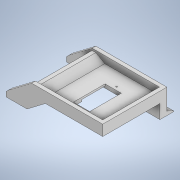
# Autodesk Inventor part: mount_for_plugs
Saved by Autodesk Inventor 2022 (Build 260153000, 153)
## iProperties
Created: 2022-01-23
Part Number: mount_for_plugs
Material: Generic
Document SubType Name: Modeling
Designer: kylem
Density: 1 g/cm^3
Appearance: Default
Author: kylem
Autodesk Inventor part; units mm, degrees
ref_plane "YZ Plane" through (0, 0, 0) normal (1, 0, 0) x (0, 1, 0)
ref_plane "XZ Plane" through (0, 0, 0) normal (0, 1, 0) x (-1, 0, 0)
sketch "Sketch1" plane through (0, 0, 0) normal (0, 1, 0) x (-1, 0, 0)
  line L0 (0, 0) -> (159.6, 0)
  line L1 (159.6, 46) -> (159.6, 118)
  line L2 (159.6, 118) -> (0, 118)
  line L3 (0, 118) -> (0, 0)
  line L4 (159.6, 118) -> (159.6, 46)
  line L5 (0, 0) -> (113, 0)
  line L6 (113, 0) -> (159.6, 46)
  line L7 (159.6, 118) -> (167.6, 118)
  line L8 (167.6, 118) -> (167.6, 46)
  line L9 (167.6, 46) -> (159.6, 46)
  line L10 (159.6, 46) -> (159.6, 118)
  line L11 (113, 0) -> (0, 0)
  line L12 (0, 0) -> (0, -8)
  line L13 (0, -8) -> (113, -8)
  line L14 (113, -8) -> (113, 0)
  line L15 (0, 0) -> (0, 10)
  line L16 (0, 10) -> (9, 10)
  circle A0 centre (9, 10) radius 2.25
  line L17 (159.6, 118) -> (159.6, 89)
  line L18 (159.6, 89) -> (149.6, 89)
  circle A1 centre (149.6, 89) radius 2.25
  line L19 (159.6, 118) -> (159.6, 0)
  dimension "d0" = 159.6
  dimension "d2" = 72
  dimension "d3" = 113
  dimension "d4" = 8
  dimension "d5" = 8
  dimension "d6" = 10
  dimension "d7" = 9
  dimension "d8" = 4.5
  dimension "d9" = 29
  dimension "d10" = 10
  dimension "d11" = 4.5
  dimension "d14" = 118
  constraints: 40 end point, 6 parallel, 5 perpendicular, 3 horizontal, 3 point on line, 2 centre point, 2 coincident, 1 collinear
  measures "d0" distance of L2.end L1.end
  measures "d2" distance of L1.start L1.end
  measures "d3" distance of L0.start L5.end
  measures "d4" distance of L1.start L8.end
  measures "d5" distance of L12.end L11.end
  measures "d6" distance of L11.end L15.end
  measures "d7" distance of L15.end L16.end
  measures "d8" diameter of A0
  measures "d9" distance of L1.end L17.end
  measures "d10" distance of L17.end L18.end
  measures "d11" diameter of A1
  measures "d14" distance of L1.end L0.end
extrude "Extrusion2" add sketch "Sketch1" along normal blind 8 contours L3 L2 L1 L6 L0 | L0 L14 L13 L12 | L1 L7 L8 L9
sketch "Sketch2" plane through (0, 8, 0) normal (0, 1, 0) x (1, 0, 0)
  line L0 (-113, 8) -> (-113, 0) projected
  line L1 (-159.6, -46) -> (-113, 0)
  line L2 (-113, 0) -> (-94.4074, 18.3532)
  line L3 (-113, 0) -> (-159.6, -46) projected
  line L4 (-113, 0) -> (-159.6, -46)
  line L5 (-159.6, -46) -> (-175.759, -61.951)
  line L6 (-175.759, -61.951) -> (-174.3006, -39.4963)
  line L7 (-174.3006, -39.4963) -> (-106.8014, 20.2158)
  line L8 (-106.8014, 20.2158) -> (-94.4074, 18.3532)
  point P0 (0, 0)
  constraints: 14 end point, 2 point on line, 1 collinear
extrude "Extrusion3" cut sketch "Sketch2" against normal blind 10
sketch "Sketch3" plane through (0, 0, 0) normal (0, -1, 0) x (1, 0, 0)
  line L0 (-167.6, 118) -> (0, 118) projected
  line L1 (-167.6, 118) -> (-167.6, 92.4)
  line L2 (-167.6, 53.897) -> (-167.6, 118) projected
  line L3 (-167.6, 92.4) -> (-128, 92.4)
  line L4 (-128, 92.4) -> (-120.5, 92.4)
  line L5 (-120.5, 92.4) -> (-120.5, 88.9)
  line L6 (-120.5, 88.9) -> (-128, 88.9)
  line L7 (-128, 88.9) -> (-128, 92.4)
  line L8 (-120.5, 88.9) -> (-120.5, 56.15)
  line L9 (-120.5, 88.9) -> (-87.75, 88.9) construction
  circle A0 centre (-120.5, 88.9) radius 1.15
  circle A1 centre (-120.5, 56.15) radius 1.15
  line L10 (-120.5, 88.9) -> (-120.5, 90.9)
  line L11 (-120.5, 88.9) -> (-120.5, 85.9)
  line L12 (-120.5, 56.15) -> (-120.5, 59.15)
  line L13 (-120.5, 59.15) -> (-115, 59.15)
  line L14 (-120.5, 85.9) -> (-126, 85.9)
  line L15 (-126, 85.9) -> (-115, 85.9)
  line L16 (-115, 85.9) -> (-115, 59.15)
  line L17 (-115, 59.15) -> (-126, 59.15)
  line L18 (-126, 59.15) -> (-126, 85.9)
  point P0 (0, 0)
  dimension "d19" = 25.6
  dimension "d20" = 39.6
  dimension "d21" = 7.5
  dimension "d22" = 3.5
  dimension "d23" = 32.75
  dimension "d24" = 90
  dimension "d25" = 2.3
  dimension "d26" = 2.3
  dimension "d29" = 2
  dimension "d30" = 3
  dimension "d31" = 3
  dimension "d32" = 5.5
  dimension "d33" = 5.5
  constraints: 34 end point, 5 horizontal, 4 parallel, 4 perpendicular, 4 point on line, 2 centre point, 2 coincident, 1 vertical
  measures "d19" distance of L0.start L1.end
  measures "d20" distance of L1.end L3.end
  measures "d21" distance of L5.end L6.end
  measures "d22" distance of L4.end L5.end
  measures "d23" distance of L5.end L8.end
  measures "d24" angle of L8 L9
  measures "d25" diameter of A0
  measures "d26" diameter of A1
  measures "d29" distance of L10.start L10.end
  measures "d30" distance of L10.start L11.end
  measures "d31" distance of L12.start L12.end
  measures "d32" distance of L12.end L13.end
  measures "d33" distance of L11.end L14.end
extrude "Extrusion4" cut sketch "Sketch3" against normal blind 5 contours A0 L5 L6 | L6 L8 A0 | A0 L8 L5 | A1
sketch "Sketch5" plane through (0, 8, 0) normal (0, 1, 0) x (1, 0, 0)
  circle A0 centre (-9, -10) radius 2.25 projected
  circle A1 centre (-149.6, -89) radius 2.25 projected
  line L0 (-9, -10) -> (-149.6, -89)
  line L1 (-149.6, -89) -> (-116.8523, -147.2827)
  line L2 (-116.8523, -147.2827) -> (-175.4275, -43.0335)
  line L3 (-149.6, -89) -> (-9, -10)
  line L4 (-79.3, -49.5) -> (-9, -10)
  line L5 (-149.6, -89) -> (-144.7015, -97.7181)
  line L6 (-116.8523, -147.2827) -> (-175.4275, -43.0335)
  line L7 (-175.4275, -43.0335) -> (-34.8275, 35.9665)
  line L8 (-34.8275, 35.9665) -> (23.7477, -68.2827)
  line L9 (23.7477, -68.2827) -> (-116.8523, -147.2827)
  circle A2 centre (-9, -10) radius 4.5 projected
  line L10 (-9, -10) -> (-4.1015, -18.7181)
  line L11 (-4.1015, -18.7181) -> (-1.6523, -23.0771)
  line L12 (-1.6523, -23.0771) -> (8.1447, -40.5133)
  line L13 (8.1447, -40.5133) -> (10.594, -44.8723)
  line L14 (-144.7015, -97.7181) -> (-142.2523, -102.0771)
  line L15 (-142.2523, -102.0771) -> (-132.4553, -119.5133)
  line L16 (-132.4553, -119.5133) -> (-130.006, -123.8723)
  line L17 (-149.6, -89) -> (-154.4985, -80.2819)
  line L18 (-154.4985, -80.2819) -> (-156.9477, -75.9229)
  line L19 (-9, -10) -> (-13.8985, -1.2819)
  line L20 (-13.8985, -1.2819) -> (-16.3477, 3.0771)
  line L21 (-167.6, -53.897) -> (-167.6, -118) projected
  line L22 (-167.6, -118) -> (0, -118)
  line L23 (0, -118) -> (0, 8)
  line L24 (0, 8) -> (-167.6, 8)
  line L25 (-167.6, 8) -> (-167.6, -118)
  line L26 (-16.3477, 3.0771) -> (-156.9477, -75.9229)
  line L27 (-154.4985, -80.2819) -> (-13.8985, -1.2819)
  line L28 (-4.1015, -18.7181) -> (-144.7015, -97.7181)
  line L29 (-142.2523, -102.0771) -> (-1.6523, -23.0771)
  line L30 (8.1447, -40.5133) -> (-132.4553, -119.5133)
  line L31 (-130.006, -123.8723) -> (10.594, -44.8723)
  line L32 (-4.1015, -18.7181) -> (7.818, -12.0208)
  line L33 (-1.6523, -23.0771) -> (4.3075, -19.7285)
  line L34 (-13.8985, -1.2819) -> (7.818, 10.9201)
  line L35 (-16.3477, 3.0771) -> (3.62, 14.2965)
  line L36 (-144.7015, -97.7181) -> (-142.2523, -102.0771)
  line L37 (-142.2523, -102.0771) -> (-178.8351, -122.6322)
  line L38 (-178.8351, -122.6322) -> (-181.2843, -118.2731)
  line L39 (-181.2843, -118.2731) -> (-144.7015, -97.7181)
  line L40 (-154.4985, -80.2819) -> (-156.9477, -75.9229)
  line L41 (-156.9477, -75.9229) -> (-183.573, -90.883)
  line L42 (-183.573, -90.883) -> (-181.1237, -95.242)
  line L43 (-181.1237, -95.242) -> (-154.4985, -80.2819)
  line L44 (0, 8) -> (-104.8957, 8) projected
  line L45 (0, 8) -> (-5, 8)
  line L46 (-5, 8) -> (-5, 3)
  line L47 (-5, 3) -> (0, 3)
  line L48 (0, 3) -> (0, 8)
  line L49 (-104.8957, 8) -> (-167.6, -53.897) projected
  line L50 (-104.8957, 8) -> (-167.6, -53.897)
  line L51 (-167.6, -53.897) -> (-164.0874, -57.4554)
  line L52 (-164.0874, -57.4554) -> (-101.3831, 4.4416)
  line L53 (-101.3831, 4.4416) -> (-104.8957, 8)
  line L54 (0, -118) -> (0, 8) projected
  line L55 (0, 3) -> (0, 8)
  line L56 (0, 8) -> (-113.2487, 8)
  line L57 (-113.2487, 8) -> (-113.2487, 3)
  line L58 (-113.2487, 3) -> (0, 3)
  line L59 (-5, 8) -> (0, 8)
  line L60 (0, 8) -> (0, -118)
  line L61 (0, -118) -> (-5, -118)
  line L62 (-5, -118) -> (-5, 8)
  line L63 (-167.6, -118) -> (0, -118) projected
  line L64 (-167.6, -118) -> (-162.6, -118)
  line L65 (-162.6, -118) -> (-162.6, -39.4397)
  line L66 (-162.6, -39.4397) -> (-167.6, -39.4397)
  line L67 (-167.6, -39.4397) -> (-167.6, -118)
  line L68 (-167.6, -118) -> (0, -118) projected
  line L69 (0, -118) -> (-186.0038, -118)
  line L70 (-186.0038, -118) -> (-186.0038, -113)
  line L71 (-186.0038, -113) -> (0, -113)
  line L72 (0, -113) -> (0, -118)
  point P0 (0, 0)
  point P1 (-162.6, -107.7748)
  point P2 (-162.6, -84.834)
  point P3 (-6.2777, 3)
  point P4 (-5, -7.9384)
  point P5 (-5, -12.0616)
  point P6 (-5, -19.2229)
  point P7 (-5, -24.9581)
  point P8 (-5, -47.899)
  point P9 (-120.8633, -113)
  point P10 (-161.6922, -113)
  point P11 (-162.6, -113.51)
  point P12 (-162.6, -113)
  point P13 (-5, -113)
  point P14 (-110.6561, -113)
  point P15 (-5, -53.6342)
  point P16 (-162.6, -79.0988)
  point P17 (-162.6, -55.9871)
  point P18 (-102.8435, 3)
  point P19 (-16.485, 3)
  point P20 (-16.3044, 3)
  dimension "d45" = 10
  dimension "d46" = 10
  dimension "d47" = 5
  dimension "d48" = 20
  dimension "d49" = 5
  dimension "d50" = 5
  dimension "d51" = 20
  dimension "d52" = 5
  dimension "d53" = 10
  dimension "d54" = 5
  dimension "d55" = 10
  dimension "d56" = 5
  dimension "d57" = 5
  dimension "d58" = 5
  dimension "d59" = 5
  dimension "d60" = 5
  dimension "d61" = 5
  constraints: 134 end point, 20 parallel, 14 point on line, 13 perpendicular, 7 collinear, 3 horizontal, 1 midpoint
  measures "d45" distance of L0.end L5.end
  measures "d46" distance of L10.start L10.end
  measures "d47" distance of L10.end L11.end
  measures "d48" distance of L11.end L12.end
  measures "d49" distance of L12.end L13.end
  measures "d50" distance of L5.end L14.end
  measures "d51" distance of L14.end L15.end
  measures "d52" distance of L15.end L16.end
  measures "d53" distance of L0.end L17.end
  measures "d54" distance of L17.end L18.end
  measures "d55" distance of L10.start L19.end
  measures "d56" distance of L19.end L20.end
  measures "d57" distance of L47.end L46.end
  measures "d58" distance of L46.end L45.end
  measures "d59" distance of L51.end L21.start
  measures "d60" distance of L66.end L65.end
  measures "d61" distance of L69.end L70.end
extrude "Extrusion7" cut sketch "Sketch3" against normal blind 7 contours L15 L16 L13 L8 | L8 L17 L18 L14
sketch "Sketch7" plane through (0, 0, 0) normal (0, -1, 0) x (1, 0, 0)
  line L0 (-167.6, 118) -> (0, 118) projected
  line L1 (0, 118) -> (-70, 118)
  line L2 (-70, 118) -> (-70, 100.4)
  line L3 (-70, 100.4) -> (-70, 18)
  circle A0 centre (-70, 100.4) radius 1.5
  circle A1 centre (-70, 18) radius 1.5
  point P0 (0, 0)
  dimension "d66" = 70
  dimension "d67" = 17.6
  dimension "d68" = 82.4
  dimension "d69" = 3
  dimension "d70" = 3
  constraints: 6 end point, 2 centre point, 2 coincident, 1 perpendicular, 1 point on line, 1 vertical
  measures "d66" distance of L0.end L1.end
  measures "d67" distance of L1.end L2.end
  measures "d68" distance of L2.end L3.end
  measures "d69" diameter of A0
  measures "d70" diameter of A1
extrude "Extrusion8" cut sketch "Sketch7" against normal blind 30
sketch "Sketch8" plane through (0, 0, 0) normal (0, -1, 0) x (1, 0, 0)
  circle A0 centre (-70, 100.4) radius 1.5 projected
  line L0 (-70, 100.4) -> (-70, 93.4)
  line L1 (-70, 93.4) -> (-52.5, 93.4)
  line L2 (-52.5, 93.4) -> (-87.5, 93.4)
  line L3 (-87.5, 93.4) -> (-87.5, 25.4)
  line L4 (-87.5, 25.4) -> (-52.5, 25.4)
  line L5 (-52.5, 25.4) -> (-52.5, 93.4)
  point P0 (0, 0)
  dimension "d73" = 7
  dimension "d74" = 17.5
  dimension "d75" = 35
  dimension "d76" = 68
  constraints: 12 end point, 2 horizontal, 2 parallel, 1 perpendicular, 1 vertical
  measures "d73" distance of L0.start L0.end
  measures "d74" distance of L0.end L1.end
  measures "d75" distance of L4.end L3.end
  measures "d76" distance of L3.end L2.end
extrude "Extrusion9" cut sketch "Sketch8" against normal blind 23 contours L1 L5 L4 L3 L2
extrude "Extrusion10" add sketch "Sketch5" along normal blind 15 contours L62 L47 L23 L32 L8 A2 | L8 L28 L62 | L8 L35 L24 L46 L34 L58 | L34 L46 L58 | L46 L34 L23 L47 | L32 L23 L33 L8 | L8 L29 L62 L28 | L26 L58 L7 L24 L8 | L8 L24 L35 | L65 L39 L21 L43 | L43 L21 L41 L65 | L46 L24 L23 L34 | L33 L23 L8 | L8 L23 L30 L62 L29 | L58 L52 L53 L24 L7 | L65 L41 L21 L2 | L2 L21 L51 L52 L65 | L65 L71 L21 L39 | L30 L23 L31 L62 | L52 L65 L49 L7 | L7 L49 L58 L52 | L58 L49 L53 L52 | L52 L51 L49 L65 | L71 L37 L65 | L65 L37 L21 L71 | L71 L30 L22 L1 | L1 L22 L65 L37 L71 | L71 L31 L22 L30 | L31 L23 L9 L62 | L65 L22 L21 L37 | L71 L9 L22 L31 | L9 L23 L71 L62 | L71 L62 L22 L9 | L71 L23 L22 L62
sketch "Sketch10" plane through (0, 0, 0) normal (0, -1, 0) x (1, 0, 0)
  line L0 (-52.5, 93.4) -> (-87.5, 93.4) projected
  line L1 (-70, 93.4) -> (-42.5, 93.4)
  line L2 (-42.5, 93.4) -> (-42.5, 75.4)
  line L3 (-42.5, 75.4) -> (-42.5, 25.4)
  line L4 (-42.5, 75.4) -> (-97.5, 75.4)
  line L5 (-97.5, 75.4) -> (-97.5, 25.4)
  line L6 (-97.5, 25.4) -> (-42.5, 25.4)
  line L7 (-42.5, 25.4) -> (-42.5, 75.4)
  point P0 (0, 0)
  point P1 (-42.5, 25.4)
  dimension "d81" = 27.5
  dimension "d82" = 18
  dimension "d83" = 50
  dimension "d84" = 55
  dimension "d87" = 50
  constraints: 14 end point, 2 parallel, 2 perpendicular, 1 collinear, 1 horizontal, 1 midpoint, 1 point on line
  measures "d81" distance of L1.start L1.end
  measures "d82" distance of L1.end L2.end
  measures "d83" distance of L2.end L3.end
  measures "d84" distance of L6.end L5.end
  measures "d87" distance of L4.end L5.end
extrude "Extrusion11" cut sketch "Sketch10" against normal blind 4
sketch "Sketch11" plane through (0, 8, 0) normal (0, 1, 0) x (1, 0, 0)
  line L0 (-162.6, -55.9871) -> (-102.8435, 3) projected
  line L1 (-162.6, -55.9871) -> (-102.8435, -55.9871)
  line L2 (-102.8435, -55.9871) -> (-102.8435, 3)
  line L3 (-102.8435, 3) -> (-162.6, 3)
  line L4 (-162.6, 3) -> (-162.6, -55.9871)
  point P0 (0, 0)
  constraints: 8 end point, 2 parallel, 1 horizontal, 1 perpendicular
extrude "Extrusion12" cut sketch "Sketch11" along normal blind 20 contours L4 L3 L0
sketch "Sketch12" plane through (0, 8, 0) normal (0, 1, 0) x (1, 0, 0)
  line L0 (0, 8) -> (-104.8957, 8) projected
  line L1 (-167.6, -53.897) -> (-104.8957, -53.897)
  line L2 (-104.8957, -53.897) -> (-104.8957, 8)
  line L3 (-104.8957, 8) -> (-167.6, 8)
  line L4 (-167.6, 8) -> (-167.6, -53.897)
  line L5 (-104.8957, 8) -> (-109.9609, 3) projected
  line L6 (-162.6, -48.9614) -> (-109.9609, 3) projected
  line L7 (-109.9609, 3) -> (-162.6, 3)
  line L8 (-162.6, 3) -> (-162.6, -48.9614)
  line L9 (-162.6, -48.9614) -> (-109.9609, -48.9614)
  line L10 (-109.9609, -48.9614) -> (-109.9609, 3)
  point P0 (0, 0)
  constraints: 16 end point, 4 parallel, 2 horizontal, 2 perpendicular
extrude "Extrusion13" add sketch "Sketch12" against normal blind 8 contours L8 L7 L6
sketch "Sketch13" plane through (0, 8, 0) normal (0, 1, 0) x (1, 0, 0)
  line L0 (-104.8957, 8) -> (-109.9609, 3) projected
  line L1 (-167.6, -53.897) -> (-167.6, -118) projected
  line L2 (-104.8957, 8) -> (-167.6, 8)
  line L3 (-167.6, 8) -> (-167.6, -53.897)
  line L4 (-167.6, -53.897) -> (-104.8957, -53.897)
  line L5 (-104.8957, -53.897) -> (-104.8957, 8)
  line L6 (-167.6, -53.897) -> (-162.6, -48.9614) projected
  line L7 (-109.9609, 3) -> (-162.6, 3)
  line L8 (-162.6, 3) -> (-162.6, -48.9614)
  line L9 (-162.6, -48.9614) -> (-109.9609, -48.9614)
  line L10 (-109.9609, -48.9614) -> (-109.9609, 3)
  point P0 (0, 0)
  constraints: 16 end point, 4 parallel, 2 horizontal, 2 perpendicular
extrude "Extrusion14" add sketch "Sketch13" along normal blind 15 contours L0 L7 L8 L6 L3 L2
extrude "Extrusion15" add sketch "Sketch13" against normal blind 8 contours L0 L7 L8 L6 L3 L2
sketch "Sketch14" plane through (0, 8, 0) normal (0, 1, 0) x (1, 0, 0)
  circle A0 centre (-9, -10) radius 2.25 projected
  circle A1 centre (-9, -10) radius 2.25
  circle A2 centre (-149.6, -89) radius 2.25 projected
  circle A3 centre (-149.6, -89) radius 2.25
  point P0 (0, 0)
  constraints: 2 centre point, 2 coincident
extrude "Extrusion16" add sketch "Sketch14" against normal blind 8
sketch "Sketch15" plane through (-162.6, 8, -3) normal (0, 0, 1) x (1, 0, 0)
  line L0 (0, 0) -> (0, 15) projected
  line L1 (0, 0) -> (187.1145, 0)
  line L2 (187.1145, 0) -> (187.1145, 32.8741)
  line L3 (187.1145, 32.8741) -> (0, 32.8741)
  line L4 (0, 32.8741) -> (0, 0)
  line L5 (0, 0) -> (-28.6153, 0)
  line L6 (-28.6153, 0) -> (-28.6153, 26.9098)
  line L7 (-28.6153, 26.9098) -> (0, 26.9098)
  line L8 (0, 26.9098) -> (0, 0)
  point P0 (162.6, -8)
  constraints: 16 end point, 4 parallel, 2 horizontal, 2 perpendicular
extrude "Extrusion17" cut sketch "Sketch15" along normal mid plane 900
sketch "Sketch16" plane through (0, 8, 0) normal (0, 1, 0) x (1, 0, 0)
  line L0 (-167.6, 8) -> (0, 8) projected
  line L1 (0, 8) -> (-167.6, 8)
  line L2 (-167.6, 8) -> (-167.6, 20)
  line L3 (-167.6, 20) -> (0, 20)
  line L4 (0, 20) -> (0, 8)
  point P0 (0, 0)
  dimension "d100" = 12
  constraints: 8 end point, 2 parallel, 1 horizontal, 1 perpendicular
  measures "d100" distance of L1.end L2.end
extrude "Extrusion18" add sketch "Sketch16" against normal blind 8
sketch "Sketch17" plane through (0, 0, 0) normal (0, -1, 0) x (1, 0, 0)
  line L0 (-167.6, 118) -> (0, 118) projected
  line L1 (-167.6, -20) -> (0, -20) projected
  line L2 (-167.6, 118) -> (-152.6, 118)
  line L3 (-152.6, 118) -> (-152.6, -20)
  line L4 (-152.6, -20) -> (-167.6, -20)
  line L5 (-167.6, -20) -> (-167.6, 118)
  point P0 (0, 0)
  dimension "d103" = 15
  constraints: 8 end point, 2 parallel, 1 horizontal, 1 perpendicular, 1 point on line
  measures "d103" distance of L3.end L4.end
extrude "Extrusion19" cut sketch "Sketch17" against normal blind 8
sketch "Sketch18" plane through (0, 0, 0) normal (0, -1, 0) x (1, 0, 0)
  line L0 (0, -20) -> (-152.6, -20) projected
  line L1 (-152.6, -20) -> (-152.6, 118) projected
  line L2 (0, -20) -> (-152.6, -20)
  line L3 (-152.6, -20) -> (-152.6, -5)
  line L4 (-152.6, -5) -> (0, -5)
  line L5 (0, -5) -> (0, -20)
  line L6 (-152.6, 118) -> (-137.6, 118)
  line L7 (-137.6, 118) -> (-137.6, -5)
  line L8 (-137.6, -5) -> (-152.6, -5)
  line L9 (-152.6, -5) -> (-152.6, 118)
  point P0 (0, 0)
  dimension "d106" = 15
  dimension "d107" = 15
  constraints: 16 end point, 4 parallel, 2 horizontal, 2 perpendicular, 2 point on line
  measures "d106" distance of L2.end L3.end
  measures "d107" distance of L7.end L8.end
extrude "Extrusion20" add sketch "Sketch18" along normal blind 30
sketch "Sketch19" plane through (-152.6, 8, -20) normal (-1, 0, 0) x (0, 0, 1)
  line L0 (138, 0) -> (138, -38) projected
  line L1 (0, -38) -> (138, -38)
  line L2 (138, -38) -> (138, -23)
  line L3 (138, -23) -> (0, -23)
  line L4 (0, -23) -> (0, -38)
  point P0 (20, -8)
  dimension "d110" = 15
  constraints: 8 end point, 2 parallel, 1 horizontal, 1 perpendicular, 1 point on line
  measures "d110" distance of L2.end L1.end
extrude "Extrusion21" add sketch "Sketch19" along normal blind 70
ref_plane "Work Plane1" through (0, 0, 49) normal (0, 0, 1) x (1, 0, 0)
sketch "Sketch21" plane through (0, 8, 0) normal (0, 1, 0) x (1, 0, 0)
  line L0 (0, 20) -> (-152.6, 20) projected
  line L1 (0, 20) -> (-8, 20)
  line L2 (-8, 20) -> (-8, 12)
  line L3 (-8, 12) -> (0, 12)
  line L4 (0, 12) -> (0, 20)
  line L5 (0, -118) -> (-152.6, -118) projected
  line L6 (-152.6, -118) -> (-144.6, -118)
  line L7 (-144.6, -118) -> (-144.6, -110)
  line L8 (-144.6, -110) -> (-152.6, -110)
  line L9 (-152.6, -110) -> (-152.6, -118)
  line L10 (-144.6, -110) -> (-8, -110)
  line L11 (-8, -110) -> (-8, 12)
  line L12 (-8, 12) -> (-144.6, 12)
  line L13 (-144.6, 12) -> (-144.6, -110)
  line L14 (0, 20) -> (-152.6, 20)
  line L15 (-152.6, 20) -> (-152.6, -118)
  line L16 (-152.6, -118) -> (0, -118)
  line L17 (0, -118) -> (0, 20)
  point P0 (0, 0)
  dimension "d116" = 8
  dimension "d117" = 8
  dimension "d118" = 8
  dimension "d119" = 8
  constraints: 32 end point, 8 parallel, 4 horizontal, 4 perpendicular
  measures "d116" distance of L3.end L2.end
  measures "d117" distance of L2.end L1.end
  measures "d118" distance of L8.end L7.end
  measures "d119" distance of L7.end L6.end
extrude "Extrusion23" add sketch "Sketch21" along normal blind 15 contours L4 L3 L2 L0 | L2 L12 L13 L8 L15 L0 | L17 L5 L7 L10 L11 L3 | L8 L7 L5 L9
sketch "Sketch22" plane through (-137.6, 0, 118) normal (0, 0, 1) x (1, 0, 0)
  line L0 (-15, -15) -> (-15, 23) projected
  line L1 (-15, -15) -> (-85, -15) projected
  line L2 (-15, 23) -> (-65, 23)
  line L3 (-65, 23) -> (-65, -15)
  line L4 (-65, -15) -> (-15, -15)
  line L5 (-15, -15) -> (-15, 23)
  line L6 (-15, 23) -> (-65, -15)
  point P0 (137.6, 0)
  dimension "d123" = 50
  constraints: 10 end point, 2 parallel, 1 horizontal, 1 perpendicular, 1 point on line
  measures "d123" distance of L4.end L3.end
extrude "Extrusion24" add sketch "Sketch22" against normal blind 8 contours L1 L6 L0
mirror "Mirror2" about plane through (0, 0, 49) normal (0, 0, 1) of "Extrusion24"
sketch "Sketch23" plane through (0, -30, 0) normal (0, -1, 0) x (1, 0, 0)
  line L0 (0, -20) -> (0, -5) projected
  line L1 (0, -20) -> (-170, -20)
  line L2 (-170, -20) -> (-170, -35)
  line L3 (-170, -35) -> (0, -35)
  line L4 (0, -35) -> (0, -20)
  point P0 (0, 0)
  dimension "d126" = 170
  dimension "d127" = 15
  constraints: 8 end point, 2 parallel, 1 horizontal, 1 perpendicular
  measures "d126" distance of L3.end L2.end
  measures "d127" distance of L2.end L1.end
extrude "Extrusion25" add sketch "Sketch23" against normal blind 8
sketch "Sketch24" plane through (-222.6, -15, 118) normal (0, 1, 0) x (1, 0, 0)
  line L0 (85, 0) -> (0, 0) projected
  line L1 (52.6, 138) -> (0, 138) projected
  line L2 (0, 0) -> (15, 0)
  line L3 (15, 0) -> (15, 138)
  line L4 (15, 138) -> (0, 138)
  line L5 (0, 138) -> (0, 0)
  point P0 (222.6, 118)
  dimension "d130" = 15
  constraints: 8 end point, 2 parallel, 1 horizontal, 1 perpendicular, 1 point on line
  measures "d130" distance of L4.end L3.end
extrude "Extrusion26" cut sketch "Sketch24" against normal blind 100
sketch "Sketch25" plane through (0, -30, 0) normal (0, -1, 0) x (1, 0, 0)
  line L0 (0, -5) -> (-137.6, -5) projected
  line L1 (0, -5) -> (-45, -5)
  line L2 (-45, -5) -> (-45, -15)
  line L3 (-45, -15) -> (0, -15)
  line L4 (0, -15) -> (0, -5)
  circle A0 centre (-45, -15) radius 2.25
  point P0 (0, 0)
  dimension "d133" = 45
  dimension "d134" = 10
  dimension "d135" = 4.5
  constraints: 8 end point, 2 parallel, 1 centre point, 1 coincident, 1 horizontal, 1 perpendicular
  measures "d133" distance of L3.end L2.end
  measures "d134" distance of L2.end L1.end
  measures "d135" diameter of A0
sketch "Sketch26" plane through (0, -30, 0) normal (0, -1, 0) x (1, 0, 0)
  line L0 (-170, -20) -> (-207.6, -20) projected
  line L1 (-207.6, -20) -> (-121.6, -20)
  line L2 (-121.6, -20) -> (-121.6, -15)
  line L3 (0, -5) -> (-137.6, -5) projected
  circle A0 centre (-121.6, -15) radius 2.25
  point P0 (0, 0)
  dimension "d136" = 86
  dimension "d137" = 5
  dimension "d138" = 4.5
  constraints: 4 end point, 1 centre point, 1 coincident, 1 collinear, 1 perpendicular
  measures "d136" distance of L0.end L1.end
  measures "d137" distance of L1.end L2.end
  measures "d138" diameter of A0
extrude "Extrusion27" cut sketch "Sketch26" against normal blind 20
extrude "Extrusion28" cut sketch "Sketch25" against normal blind 20 contours A0 L3 L2 | L2 L3 A0
sketch "Sketch27" plane through (0, -30, 0) normal (0, -1, 0) x (1, 0, 0)
  circle A0 centre (-121.6, -15) radius 2.25 projected
  line L0 (-121.6, -15) -> (-101.6, -15)
  line L1 (-101.6, -15) -> (-81.6, -15)
  circle A1 centre (-45, -15) radius 2.25 projected
  line L2 (-45, -15) -> (-65, -15)
  circle A2 centre (-101.6, -15) radius 2.25
  circle A3 centre (-81.6, -15) radius 2.25
  circle A4 centre (-65, -15) radius 2.25
  point P0 (0, 0)
  dimension "d143" = 20
  dimension "d144" = 20
  dimension "d145" = 20
  dimension "d146" = 4.5
  dimension "d147" = 4.5
  dimension "d148" = 4.5
  constraints: 6 end point, 3 centre point, 3 coincident, 2 horizontal, 1 point on line
  measures "d143" distance of L0.start L0.end
  measures "d144" distance of L0.end L1.end
  measures "d145" distance of L2.start L2.end
  measures "d146" diameter of A2
  measures "d147" diameter of A3
  measures "d148" diameter of A4
extrude "Extrusion29" cut sketch "Sketch27" against normal blind 20 contours A2 L1 L0 | L0 L1 A2 | A3 | A4
sketch "Sketch28" plane through (-202.6, -15, 110) normal (0, 1, 0) x (1, 0, 0)
  line L0 (0, 122) -> (50, 122) projected
  line L1 (50, 122) -> (-30.0077, 122)
  line L2 (-30.0077, 122) -> (-30.0077, 0)
  line L3 (-30.0077, 0) -> (50, 0)
  line L4 (50, 0) -> (50, 122)
  point P0 (202.6, 110)
  constraints: 8 end point, 2 parallel, 1 horizontal, 1 perpendicular
extrude "Extrusion30" cut sketch "Sketch28" against normal blind 100
sketch "Sketch29" plane through (-137.6, 0, 118) normal (1, 0, 0) x (0, 0, -1)
  line L0 (0, 0) -> (0, -30) projected
  line L1 (8, 23) -> (8, -30) projected
  line L2 (0, 0) -> (8, 0)
  line L3 (8, 0) -> (8, -30)
  line L4 (8, -30) -> (0, -30)
  line L5 (0, -30) -> (0, 0)
  line L6 (0, -30) -> (8, -30) projected
  line L7 (8, -30) -> (123, -30)
  line L8 (123, -30) -> (123, 0)
  line L9 (123, 0) -> (8, 0)
  line L10 (8, 0) -> (8, -30)
  point P0 (118, 0)
  constraints: 16 end point, 4 parallel, 2 horizontal, 2 perpendicular
extrude "Extrusion31" cut sketch "Sketch29" against normal blind 100 contours L9 L8 L7 L1
sketch "Sketch30" plane through (-137.6, 0, 118) normal (0, 0, 1) x (1, 0, 0)
  line L0 (-15, 23) -> (-15, -30) projected
  line L1 (-15, 23) -> (-15, -15)
  line L2 (-15, 23) -> (-15, -30) projected
  line L3 (-70, -15) -> (-65, -15) projected
  line L4 (-65, -15) -> (-15, -15)
  line L5 (0, 0) -> (0, -30) projected
  line L6 (0, -30) -> (-25, -30)
  line L7 (-25, -30) -> (-25, -11)
  line L8 (-25, -11) -> (0, -11)
  line L9 (0, -11) -> (0, -30)
  line L10 (0, -11) -> (-25, -30)
  point P0 (137.6, 0)
  point P1 (-15, 0)
  dimension "d158" = 25
  dimension "d159" = 19
  constraints: 14 end point, 2 parallel, 2 perpendicular, 1 horizontal, 1 point on line
  measures "d158" distance of L7.end L8.end
  measures "d159" distance of L6.end L7.end
extrude "Extrusion32" cut sketch "Sketch30" against normal blind 10 contours L5 L6 L0 L10 | L0 L6 L10
chamfer "Chamfer3" distance 7 angle 60 1 edges at (-85, -22, -35) measured on face at (-113.3333, -24.6667, -35)
chamfer "Chamfer4" distance 5 angle 45 2 edges at (-207.6, -15, -16) (-207.6, -15, 114)
chamfer "Chamfer5" distance 7 angle 75 1 edges at (-152.6, -15, -5) measured on face at (-152.6, 15.3333, 31)
chamfer "Chamfer6" distance 11 angle 45 1 edges at (-137.6, -11, 114)
sketch "Sketch31" plane through (0, 0, 118) normal (0, 0, 1) x (1, 0, 0)
  line L0 (-162.6, -30) -> (-207.6, -30) projected
  line L1 (-162.6, -30) -> (-146.3578, -17.6559)
  line L2 (-146.3578, -17.6559) -> (-103.4655, 14.9422)
  line L3 (-115, 0) -> (-126, 0) projected
  line L4 (-137.6, 0) -> (-146.3578, -17.6559) projected
  line L5 (-123.1263, 0) -> (-137.6, 0)
  line L6 (-137.6, 0) -> (-146.3578, -17.6559)
  line L7 (-146.3578, -17.6559) -> (-123.1263, 0)
  line L8 (-137.6, 0) -> (-152.6, 0) projected
  line L9 (-137.6, 0) -> (-123.1263, 0)
  point P0 (0, 0)
  constraints: 12 end point, 3 point on line, 1 collinear, 1 horizontal
extrude "Extrusion33" add sketch "Sketch31" against normal blind 8
sketch "Sketch32" plane through (0, 23, 0) normal (0, 1, 0) x (1, 0, 0)
  line L0 (-144.6, 12) -> (-144.6, -110) projected
  line L1 (-152.6, -110) -> (-152.6, -118) projected
  line L2 (-144.6, 12) -> (-152.6, 12)
  line L3 (-152.6, 12) -> (-152.6, -110)
  line L4 (-152.6, -110) -> (-144.6, -110)
  line L5 (-144.6, -110) -> (-144.6, 12)
  point P0 (0, 0)
  constraints: 8 end point, 2 parallel, 1 horizontal, 1 perpendicular
extrude "Extrusion34" cut sketch "Sketch32" against normal blind 4
chamfer "Chamfer7" distance 11 angle 60 1 edges at (-144.6, 8, 49) measured on face at (-144.6, 11.6667, 69.3333)
body "Solid2"
